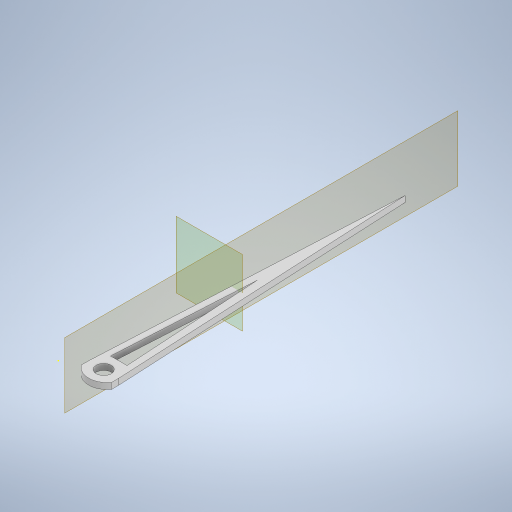
# Autodesk Inventor part: arm_v2(arm-point)
Saved by Autodesk Inventor 2024.3 (Build 283343000, 343)
## iProperties
Created: 2024-07-09
Part Number: arm_v2(arm-point)
Material: Ogólny
Document SubType Name: Modeling
Designer: User
Density: 1 g/cm^3
Appearance: Domyślna
Author: User
Autodesk Inventor part; units mm, degrees
ref_plane "YZ Plane" through (0, 0, 0) normal (1, 0, 0) x (0, 1, 0)
ref_plane "XZ Plane" through (0, 0, 0) normal (0, 1, 0) x (-1, 0, 0)
ref_plane "XY Plane" through (0, 0, 0) normal (0, 0, 1) x (1, 0, 0)
sketch "Szkic3" plane through (0, 0, 0) normal (0, 1, 0) x (-1, 0, 0)
  line L0 (0, 0) -> (10, 0)
  line L1 (10, 0) -> (10, -50)
  line L2 (10, -50) -> (0, -50)
  line L3 (0, -50) -> (0, 0)
  circle A0 centre (5, -5) radius 2.5
  arc A1 (10, -2.5) -> (0, -2.5) centre (5, -6.25) ccw
  line L4 (8, -50) -> (2, -50)
  line L5 (2, -50) -> (2, -10)
  line L6 (2, -10) -> (8, -10)
  line L7 (8, -10) -> (8, -50)
  line L8 (2, -10) -> (8, -16)
  line L9 (2, -10) -> (10.4853, -10) construction
  line L10 (8, -16) -> (8, -18)
  line L11 (8, -18) -> (2, -12)
  line L12 (2, -10) -> (2, -12)
  line L13 (8, -18) -> (8, -22)
  line L14 (2, -16) -> (8, -22)
  line L15 (8, -24) -> (2, -18)
  line L16 (8, -16) -> (8, -14)
  line L17 (8, -24) -> (8, -26)
  line L18 (2, -20) -> (8, -26)
  line L19 (8, -28) -> (2, -22)
  line L20 (8, -28) -> (8, -32)
  line L21 (2, -26) -> (8, -32)
  line L22 (8, -34) -> (2, -28)
  line L23 (8, -34) -> (8, -36)
  line L24 (2, -26) -> (8, -32)
  line L25 (8, -34) -> (2, -28)
  line L26 (8, -34) -> (8, -38)
  line L27 (2, -32) -> (8, -38)
  line L28 (8, -40) -> (2, -34)
  line L29 (8, -40) -> (8, -42)
  line L30 (2, -32) -> (8, -38)
  line L31 (8, -40) -> (2, -34)
  line L32 (8, -40) -> (8, -44)
  line L33 (2, -38) -> (8, -44)
  line L34 (8, -46) -> (2, -40)
  line L35 (8, -46) -> (8, -48)
  line L36 (2, -38) -> (8, -44)
  line L37 (8, -46) -> (2, -40)
  line L38 (8, -46) -> (8, -50)
  line L39 (8, -46) -> (8, -48)
  line L40 (8, -48) -> (2, -42)
  line L41 (2, -42) -> (2, -44)
  line L42 (2, -44) -> (8, -50)
  line L43 (7, -49) -> (2, -49)
  circle A2 centre (5, -5) radius 3.25
  dimension "d9" = 10
  dimension "d10" = 50
  dimension "d11" = 5
  dimension "d12" = 6
  dimension "d13" = 40
  dimension "d14" = 45
  dimension "d15" = 2
  dimension "d16" = 4
  dimension "d17" = 2
  dimension "d18" = 2
  dimension "d19" = 2
  dimension "d20" = 2
  dimension "d21" = 4
  dimension "d22" = 2
  dimension "d23" = 2
  dimension "d24" = 2
  dimension "d25" = 4
  dimension "d26" = 2
  dimension "d27" = 2
  dimension "d28" = 2
  dimension "d29" = 4
  dimension "d30" = 2
  dimension "d32" = 2
  dimension "d36" = 2
  dimension "d37" = 2
  dimension "d42" = 6.5
  constraints: 88 end point, 14 point on line, 13 parallel, 3 centre point, 3 horizontal, 3 perpendicular, 2 collinear, 2 point on circle, 1 coincident, 1 equal length
  measures "d9" distance of L1.end L2.end
  measures "d10" distance of L0.end L1.end
  measures "d11" diameter of A0
  measures "d12" distance of L5.end L6.end
  measures "d13" distance of L4.end L5.end
  measures "d14" angle of L8 L9
  measures "d15" distance of L8.end L10.end
  measures "d16" distance of L10.end L13.end
  measures "d17" distance of L14.end L15.start
  measures "d18" distance of L8.end L16.end
  measures "d19" distance of L15.start L17.end
  measures "d20" distance of L18.end L20.start
  measures "d21" distance of L20.start L20.end
  measures "d22" distance of L21.end L23.start
  measures "d23" distance of L23.start L23.end
  measures "d24" distance of L24.end L26.start
  measures "d25" distance of L26.start L26.end
  measures "d26" distance of L27.end L29.start
  measures "d27" distance of L29.start L29.end
  measures "d28" distance of L30.end L32.start
  measures "d29" distance of L32.start L32.end
  measures "d30" distance of L33.end L35.start
  measures "d32" distance of L36.end L38.start
  measures "d36" distance of L38.start L35.end
  measures "d37" distance of L40.end L41.end
  measures "d42" diameter of A2
extrude "Wyciągnięcie proste2" add sketch "Szkic3" against normal blind 2 contours A1 L1 L2 L7 L6 L5 L3 | L5 L43 L42 L2 | L42 L5 L40 L7 | L34 L5 L33 L7 | L28 L5 L27 L7 | L5 L21 L7 L22 | L5 L18 L7 L19 | L5 L14 L7 L15 | L5 L8 L7 L11 | A2
ref_plane "Płaszczyzna konstrukcyjna1" through (0, 0, -50) normal (0, 0, -1) x (-1, 0, 0)
mirror "Odbij1" about plane through (0, 0, -50) normal (0, 0, -1) of "Wyciągnięcie proste2"
sketch "Szkic4" plane through (0, 0, 0) normal (0, 1, 0) x (1, 0, 0)
  line L0 (-7.5, 91.0504) -> (-2.5, 91.0504)
  line L1 (-2.5, 91.0504) -> (-2.5, 98.6571)
  line L2 (-2.5, 98.6571) -> (-7.5, 98.6571)
  line L3 (-7.5, 98.6571) -> (-7.5, 91.0504)
  point P0 (0, 0)
  constraints: 8 end point, 2 parallel, 1 horizontal, 1 perpendicular
extrude "Wyciągnięcie proste3" cut sketch "Szkic4" against normal blind 2
sketch "Szkic5" plane through (0, 0, 0) normal (0, 1, 0) x (1, 0, 0)
  line L0 (-10, 2.5) -> (-10, 97.5) projected
  line L1 (-10, 97.5) -> (-10, 67.5)
  line L2 (-10, 67.5) -> (-13, 67.5)
  line L3 (-13, 67.5) -> (-13, 97.5)
  line L4 (-13, 97.5) -> (-10, 97.5)
  arc A0 (0, 97.5) -> (-10, 97.5) centre (-5, 93.75) ccw projected
  line L5 (-5, 100) -> (-5, 49.8742)
  line L6 (-5, 100) -> (45.1258, 100) construction
  line L7 (-13, 67.5) -> (-10, 62.3038)
  line L8 (-13, 67.5) -> (-7, 67.5) construction
  line L9 (-10, 62.3038) -> (-10, 67.5)
  line L10 (0, 2.5) -> (0, 97.5)
  line L11 (0, 67.5) -> (3, 67.5)
  line L12 (3, 67.5) -> (3, 97.5)
  line L13 (3, 97.5) -> (0, 97.5)
  line L14 (3, 67.5) -> (0, 62.3038)
  arc A1 (3, 97.5) -> (-13, 97.5) centre (-5, 94.4495) ccw
  point P0 (0, 0)
  dimension "d43" = 30
  dimension "d44" = 3
  dimension "d45" = 90
  dimension "d46" = 60
  constraints: 28 end point, 5 symmetric about line, 3 perpendicular, 3 point on circle, 2 equal length, 2 horizontal, 2 point on line, 1 centre point, 1 vertical
  measures "d43" distance of L0.end L1.end
  measures "d44" distance of L1.end L2.end
  measures "d45" angle of L5 L6
  measures "d46" angle of L7 L8
extrude "Wyciągnięcie proste4" add sketch "Szkic5" against normal blind 2
sketch "Szkic6" plane through (0, 0, 0) normal (0, 1, 0) x (1, 0, 0)
  line L0 (-10, 62.3038) -> (-10, 2.5) projected
  line L1 (-10, 62.3038) -> (-10, 97.356)
  line L2 (-10, 97.356) -> (0, 97.356)
  line L3 (0, 97.356) -> (0, 62.3038)
  line L4 (0, 62.3038) -> (-10, 62.3038)
  point P0 (0, 0)
  constraints: 8 end point, 3 perpendicular, 1 vertical
extrude "Wyciągnięcie proste5" cut sketch "Szkic6" against normal blind 2
sketch "Szkic7" plane through (0, 0, 0) normal (0, 1, 0) x (1, 0, 0)
  line L0 (-10, 62.3038) -> (-8, 62.3038) projected
  line L1 (-10, 62.3038) -> (-10, 67.4287)
  line L2 (-10, 62.3038) -> (-10, 97.356) projected
  line L3 (-10, 67.4287) -> (0, 67.4287)
  line L4 (0, 62.3038) -> (0, 97.356) projected
  line L5 (0, 62.3038) -> (0, 67.4287)
  line L6 (0, 62.3038) -> (-2, 62.3038) projected
  line L7 (-10, 2.5) -> (-10, 62.3038) projected
  line L8 (0, 62.3038) -> (-10, 62.3038)
  line L9 (-10, 62.3038) -> (-10, 61.2351)
  line L10 (-10, 61.2351) -> (0, 61.2351)
  line L11 (0, 61.2351) -> (0, 62.3038)
  line L12 (-10, 61.2351) -> (0, 61.2351)
  line L13 (0, 2.5) -> (0, 62.3038) projected
  line L14 (0, 61.2351) -> (0, 67.4287)
  line L15 (0, 67.4287) -> (-10, 67.4287)
  line L16 (-10, 61.2351) -> (-10, 67.4287)
  point P0 (0, 0)
  constraints: 22 end point, 5 collinear, 4 point on line, 3 perpendicular, 1 horizontal
extrude "Wyciągnięcie proste6" add sketch "Szkic7" against normal blind 2
sketch "Szkic8" plane through (0, 0, 0) normal (0, 1, 0) x (1, 0, 0)
  line L0 (-7.5, 97.356) -> (-10, 97.356) projected
  line L1 (-10, 97.356) -> (-11, 97.356)
  line L2 (-11, 97.356) -> (-11, 67.4287)
  line L3 (-11, 67.4287) -> (-10, 67.4287)
  line L4 (-10, 67.4287) -> (-10, 97.356)
  line L5 (0, 97.356) -> (1, 97.356)
  line L6 (1, 97.356) -> (1, 67.4287)
  line L7 (1, 67.4287) -> (0, 67.4287)
  line L8 (0, 67.4287) -> (0, 97.356)
  line L9 (-11, 67.4287) -> (1, 67.4287)
  line L10 (1, 67.4287) -> (1, 72.7222)
  line L11 (1, 72.7222) -> (-11, 72.7222)
  line L12 (-11, 72.7222) -> (-11, 67.4287)
  point P0 (0, 0)
  point P1 (0, 72.7222)
  point P2 (-10, 72.7222)
  dimension "d53" = 1
  dimension "d54" = 1
  constraints: 24 end point, 6 parallel, 3 horizontal, 3 perpendicular, 3 point on line
  measures "d53" distance of L3.end L2.end
  measures "d54" distance of L6.end L7.end
extrude "Wyciągnięcie proste7" cut sketch "Szkic8" against normal blind 2 contours L4 L11 L2 L1 | L8 L5 L6 L11
sketch "Szkic9" plane through (0, 0, 0) normal (0, 1, 0) x (1, 0, 0)
  line L0 (-10, 72.7222) -> (0, 72.7222)
  line L1 (0, 72.7222) -> (0, 67.3617)
  line L2 (0, 67.3617) -> (-10, 67.3617)
  line L3 (-10, 67.3617) -> (-10, 72.7222)
  point P0 (0, 0)
  constraints: 8 end point, 2 parallel, 1 horizontal, 1 perpendicular
extrude "Wyciągnięcie proste8" add sketch "Szkic9" against normal blind 2
sketch "Szkic10" plane through (0, 0, 0) normal (0, 1, 0) x (1, 0, 0)
  point P0 (0, 0)
split "Podział1" plane through (0, 0, -50) removes the side toward (0, 0, -1)
sketch "Szkic11" plane through (0, 0, 0) normal (0, 1, 0) x (1, 0, 0)
  line L0 (-10, 2.5) -> (-10, 50) projected
  line L1 (-10, 50) -> (0, 50)
  line L2 (0, 50) -> (0, 100)
  line L3 (0, 100) -> (-10, 100)
  line L4 (-10, 100) -> (-10, 50)
  line L5 (-10, 100) -> (0, 100)
  line L6 (0, 100) -> (0, 124.634)
  line L7 (0, 124.634) -> (-10, 124.634)
  line L8 (-10, 124.634) -> (-10, 100)
  line L9 (-10, 124.634) -> (-11, 124.634)
  line L10 (-11, 124.634) -> (-11, 100)
  line L11 (-11, 100) -> (-10, 100)
  line L12 (-10, 100) -> (-10, 124.634)
  line L13 (0, 124.634) -> (1, 124.634)
  line L14 (1, 124.634) -> (1, 100)
  line L15 (1, 100) -> (0, 100)
  line L16 (0, 100) -> (0, 124.634)
  line L17 (-11, 100) -> (-9, 100) construction
  line L18 (1, 100) -> (3, 100) construction
  line L19 (-11, 124.634) -> (1, 124.634)
  line L20 (1, 124.634) -> (1, 126.634)
  line L21 (1, 126.634) -> (-11, 126.634)
  line L22 (-11, 126.634) -> (-11, 124.634)
  line L23 (-11, 100) -> (-12, 100)
  line L24 (-12, 100) -> (-12, 126.634)
  line L25 (-12, 126.634) -> (-11, 126.634)
  line L26 (-11, 126.634) -> (-11, 100)
  line L27 (1, 126.634) -> (2, 126.634)
  line L28 (2, 126.634) -> (2, 100)
  line L29 (2, 100) -> (1, 100)
  line L30 (1, 100) -> (1, 126.634)
  line L31 (-12, 100) -> (-10, 96.5359)
  line L32 (-12, 100) -> (-8, 100) construction
  line L33 (2, 100) -> (0, 96.5359)
  line L34 (2, 100) -> (6, 100) construction
  line L35 (-10, 124.634) -> (-10.5, 124.634)
  line L36 (-10.5, 124.634) -> (-10.5, 100)
  line L37 (0.5, 100) -> (0.5, 124.634)
  line L38 (0.75, 100) -> (0.75, 124.634)
  line L39 (-11, 100) -> (-10.75, 100)
  line L40 (-10.75, 100) -> (-10.75, 124.634)
  point P0 (0, 0)
  dimension "d59" = 10
  dimension "d60" = 50
  dimension "d61" = 10
  dimension "d62" = 24.634
  dimension "d63" = 1
  dimension "d64" = 1
  dimension "d67" = 2
  dimension "d68" = 1
  dimension "d69" = 1
  dimension "d70" = 60
  dimension "d71" = 120
  dimension "d90" = 0.5
  dimension "d107" = 0.25
  constraints: 80 end point, 17 parallel, 11 horizontal, 11 point on line, 8 perpendicular, 2 equal length, 2 midpoint
  measures "d59" distance of L3.end L2.end
  measures "d60" distance of L2.end L1.end
  measures "d61" distance of L7.end L6.end
  measures "d62" distance of L6.end L5.end
  measures "d63" distance of L11.end L10.end
  measures "d64" distance of L14.end L15.end
  measures "d67" distance of L20.end L19.end
  measures "d68" distance of L24.end L25.end
  measures "d69" distance of L28.end L29.end
  measures "d70" angle of L31 L32
  measures "d71" angle of L33 L34
  measures "d90" distance of L7.end L35.end
  measures "d107" distance of L10.end L39.end
extrude "Wyciągnięcie proste9" add sketch "Szkic11" against normal blind 2 contours L4 L3 L2 L1 | L31 L23 L11 L4 | L2 L15 L29 L33 | L24 L25 L22 L10 L23 | L29 L14 L20 L27 L28 | L9 L22 L21 L20 L13 L7
sketch "Szkic12" plane through (0, 0, 0) normal (0, 1, 0) x (1, 0, 0)
  line L0 (-8, 51.0298) -> (-2, 51.0298)
  line L1 (-2, 51.0298) -> (-2, 96.6875)
  line L2 (-2, 96.6875) -> (-8, 96.6875)
  line L3 (-8, 96.6875) -> (-8, 51.0298)
  line L4 (-8, 51.0298) -> (-2, 54.4939)
  line L5 (-8, 51.0298) -> (-1.0718, 51.0298) construction
  line L6 (-2, 54.4939) -> (-2, 59.4939)
  line L7 (-2, 59.4939) -> (-8, 56.0298)
  line L8 (-8, 51.0298) -> (-8, 56.0298)
  line L9 (-8, 56.0298) -> (-8, 61.0298)
  line L10 (-8, 61.0298) -> (-2, 64.4939)
  line L11 (-2, 64.4939) -> (-2, 69.4939)
  line L12 (-2, 69.4939) -> (-8, 66.0298)
  line L13 (-8, 61.0298) -> (-8, 66.0298)
  line L14 (-8, 66.0298) -> (-2, 69.4939)
  line L15 (-2, 74.4939) -> (-8, 71.0298)
  line L16 (-8, 76.0298) -> (-2, 79.4939)
  line L17 (-2, 84.4939) -> (-8, 81.0298)
  line L18 (-8, 71.0298) -> (-2, 74.4939)
  line L19 (-2, 79.4939) -> (-8, 76.0298)
  line L20 (-8, 81.0298) -> (-2, 84.4939)
  line L21 (-2, 89.4939) -> (-8, 86.0298)
  line L22 (-8, 76.0298) -> (-2, 79.4939)
  line L23 (-2, 84.4939) -> (-8, 81.0298)
  line L24 (-8, 86.0298) -> (-2, 89.4939)
  line L25 (-2, 94.4939) -> (-8, 91.0298)
  point P0 (0, 0)
  dimension "d74" = 30
  dimension "d75" = 5
  dimension "d76" = 5
  dimension "d77" = 5
  dimension "d78" = 5
  dimension "d79" = 5
  dimension "d80" = 5
  dimension "d81" = 5
  dimension "d82" = 5
  dimension "d83" = 5
  dimension "d84" = 5
  dimension "d85" = 5
  dimension "d86" = 5
  constraints: 52 end point, 7 point on line, 6 parallel, 2 collinear, 2 horizontal, 1 equal length, 1 perpendicular
  measures "d74" angle of L5 L4
  measures "d75" distance of L4.end L6.end
  measures "d76" distance of L7.end L9.end
  measures "d77" distance of L10.end L11.end
  measures "d78" distance of L14.end L15.start
  measures "d79" distance of L15.end L16.start
  measures "d80" distance of L16.end L17.start
  measures "d81" distance of L18.end L19.start
  measures "d82" distance of L19.end L20.start
  measures "d83" distance of L20.end L21.start
  measures "d84" distance of L22.end L23.start
  measures "d85" distance of L23.end L24.start
  measures "d86" distance of L24.end L25.start
extrude "Wyciągnięcie proste10" cut sketch "Szkic12" against normal blind 2 contours L3 L7 L1 L4 | L3 L12 L1 L10 | L3 L16 L1 L15 | L3 L21 L1 L17 | L3 L2 L1 L25
sketch "Szkic14" plane through (0, 0, 0) normal (0, 1, 0) x (1, 0, 0)
  arc A0 (5, 2.5) -> (15, 2.5) centre (10, 6.2465) ccw
  circle A1 centre (10, 5) radius 2.5
  line L0 (5, 2.5) -> (5, 5)
  line L1 (15, 2.5) -> (15, 5)
  line L2 (5, 5) -> (10, 104.8749)
  line L3 (10, 104.8749) -> (15, 5)
  line L4 (5.1827, 8.65) -> (14.8173, 8.65)
  line L5 (6.9979, 8.65) -> (12.6647, 8.65) construction
  line L6 (5.1827, 8.65) -> (7.1827, 8.65)
  line L7 (14.8173, 8.65) -> (12.8173, 8.65)
  line L8 (12.8173, 8.65) -> (9.8313, 56.0603)
  line L9 (9.8313, 56.0603) -> (7.1827, 8.65)
  line L10 (7.2581, 10) -> (12.7322, 10)
  point P0 (0, 0)
  dimension "d91" = 10
  dimension "d92" = 5
  dimension "d93" = 100
  dimension "d103" = 2
  dimension "d104" = 2
  constraints: 22 end point, 7 point on line, 3 horizontal, 2 centre point, 2 point on circle, 2 vertical
  measures "d91" distance of L0.start L1.start
  measures "d92" diameter of A1
  measures "d93" distance of L0.end L2.end
  measures "d103" distance of L4.start L6.end
  measures "d104" distance of L4.end L7.end
extrude "Wyciągnięcie proste11" add sketch "Szkic14" against normal blind 2 contours L0 L2 L4 L3 L1 A0 | L2 L3 L4 L8 L9 | L9 L10 L8 L4
sketch "Szkic15" plane through (0, 0, 0) normal (0, 1, 0) x (1, 0, 0)
  line L0 (-8, 91.0298) -> (-8, 96.6875) projected
  line L1 (-2, 10) -> (-8, 10) projected
  line L2 (-8, 96.6875) -> (-2, 96.6875)
  line L3 (-2, 96.6875) -> (-2, 10)
  line L4 (-2, 10) -> (-8, 10)
  line L5 (-8, 10) -> (-8, 96.6875)
  point P0 (0, 0)
  constraints: 8 end point, 2 parallel, 1 horizontal, 1 perpendicular
extrude "Wyciągnięcie proste12" cut sketch "Szkic15" against normal blind 2
sketch "Szkic17" plane through (0, 0, 0) normal (0, 1, 0) x (1, 0, 0)
  line L0 (-2, 96.6875) -> (-8, 96.6875) projected
  line L1 (-8, 96.6875) -> (-8.5, 96.6875)
  line L2 (-8.5, 96.6875) -> (-7.5, 96.6875)
  line L3 (-2, 96.6875) -> (-2.5, 96.6875)
  line L4 (-2.5, 96.6875) -> (-1.5, 96.6875)
  line L5 (-8, 9.9943) -> (-8.5, 9.9943)
  line L6 (-8.5, 9.9943) -> (-7.5, 9.9943)
  line L7 (-2, 10) -> (-8, 10) projected
  line L8 (-2, 10) -> (-1.5, 10)
  line L9 (-1.5, 10) -> (-2.5, 10)
  line L10 (-1.5, 10) -> (-7.5, 96.6875)
  line L11 (-8.5, 96.6875) -> (-2.5, 10)
  line L12 (-7.5, 9.9943) -> (-1.5, 96.6875)
  line L13 (-2.5, 96.6875) -> (-8.5, 9.9943)
  point P0 (0, 0)
  point P1 (-4.9999, 60.5665)
  point P2 (-5.4999, 53.3423)
  point P3 (-4.9999, 46.1181)
  point P4 (-4.4999, 53.3423)
  dimension "d121" = 0.5
  dimension "d122" = 1
  dimension "d123" = 0.5
  dimension "d124" = 1
  dimension "d125" = 0.5
  dimension "d126" = 1
  dimension "d127" = 0.5
  dimension "d128" = 1
  constraints: 24 end point, 5 point on line, 2 horizontal, 1 collinear
  measures "d121" distance of L0.end L1.end
  measures "d122" distance of L1.end L2.end
  measures "d123" distance of L0.start L3.end
  measures "d124" distance of L3.end L4.end
  measures "d125" distance of L5.start L5.end
  measures "d126" distance of L5.end L6.end
  measures "d127" distance of L7.start L8.end
  measures "d128" distance of L8.end L9.end
extrude "Wyciągnięcie proste14" add sketch "Szkic17" against normal blind 2 contours L4 L12 L10 L13 L0 | L10 L13 L11 L1 L0 | L10 L12 L11 L13 | L10 L8 L7 L11 L12 | L11 L12 L6 L5 L13
ref_plane "Płaszczyzna konstrukcyjna5" through (3.75, 0, -2.5) normal (-1, 0, 0) x (0, -1, 0)
ref_plane "Płaszczyzna konstrukcyjna4" through (0, 0, -2.5) normal (-1, 0, 0) x (0, -1, 0)
split "Podział2" plane through (3.75, 0, -2.5) removes the side toward (-1, 0, 0)
split "Podział3" plane through (3.75, 0, -2.5) removes the side toward (-1, 0, 0)
sketch "Szkic18" plane through (3.75, 0, -2.5) normal (-1, 0, 0) x (0, -1, 0)
  line L0 (-7.6237, -125.0024) -> (12.1257, -125.0024)
  line L1 (12.1257, -125.0024) -> (12.1257, 3.8459)
  line L2 (12.1257, 3.8459) -> (-7.6237, 3.8459)
  line L3 (-7.6237, 3.8459) -> (-7.6237, -125.0024)
  point P0 (0, 2.5)
  constraints: 8 end point, 2 parallel, 1 horizontal, 1 perpendicular
extrude "Wyciągnięcie proste15" cut sketch "Szkic18" along normal blind 70
